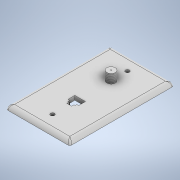
# Autodesk Inventor part: ethernet_coax_plug
Saved by Autodesk Inventor 2022 (Build 260153000, 153)
## iProperties
Created: 2022-01-23
Part Number: ethernet_coax_plug
Material: Generic
Document SubType Name: Modeling
Designer: kylem
Density: 1 g/cm^3
Appearance: Default
Author: kylem
Autodesk Inventor part; units mm, degrees
ref_plane "YZ Plane" through (0, 0, 0) normal (1, 0, 0) x (0, 1, 0)
ref_plane "XZ Plane" through (0, 0, 0) normal (0, 1, 0) x (-1, 0, 0)
ref_plane "XY Plane" through (0, 0, 0) normal (0, 0, 1) x (1, 0, 0)
sketch "Sketch1" plane through (0, 0, 0) normal (0, 1, 0) x (-1, 0, 0)
  line L0 (0, 0) -> (70, 0)
  line L1 (70, 0) -> (70, -114.4)
  line L2 (70, -114.4) -> (0, -114.4)
  line L3 (0, -114.4) -> (0, 0)
  dimension "d0" = 70
  dimension "d1" = 114.4
  constraints: 8 end point, 2 parallel, 1 horizontal, 1 perpendicular
  measures "d0" distance of L1.end L2.end
  measures "d1" distance of L0.end L1.end
extrude "Extrusion1" add sketch "Sketch1" along normal blind 4.65
sketch "Sketch2" plane through (0, 4.65, 0) normal (0, 1, 0) x (1, 0, 0)
  line L0 (-70, 0) -> (0, 0) projected
  line L1 (0, 0) -> (-35, 0)
  line L2 (-35, 0) -> (-35, 16)
  circle A0 centre (-35, 16) radius 2.125
  line L3 (0, 0) -> (0, 114.4) projected
  line L4 (0, 0) -> (0, 114.4)
  line L5 (0, 57.2) -> (13.6816, 57.2)
  circle A1 centre (-35, 98.4) radius 2.125
  dimension "d4" = 35
  dimension "d5" = 16
  dimension "d6" = 90
  dimension "d7" = 4.25
  constraints: 8 end point, 2 centre point, 2 midpoint, 1 coincident, 1 collinear, 1 horizontal, 1 perpendicular, 1 symmetric about line, 1 other
  measures "d4" distance of L0.end L1.end
  measures "d5" distance of L1.end L2.end
  measures "d6" angle of L1 L2
  measures "d7" diameter of A0
extrude "Extrusion2" cut sketch "Sketch2" against normal blind 10
fillet "Fillet1" radius 4.65 4 edges at (-35, 4.65, -114.4) (0, 4.65, -57.2) (-35, 4.65, 0) (-70, 4.65, -57.2)
fillet "Fillet2" radius 2 4 edges at (-1.3618, 3.2882, -1.3618) (-68.6382, 3.2882, -1.3618) (-68.6382, 3.2882, -113.0382) (-1.3618, 3.2882, -113.0382)
sketch "Sketch3" plane through (0, 4.65, 0) normal (0, 1, 0) x (1, 0, 0)
  line L0 (0, 0) -> (0, 34.4)
  line L1 (0, 2) -> (0, 112.4) projected
  line L2 (0, 34.4) -> (-70, 34.4)
  line L3 (-70, 112.4) -> (-70, 2) projected
  line L4 (-35, 34.4) -> (-29.125, 34.4)
  line L5 (-29.125, 34.4) -> (-40.875, 34.4)
  line L6 (-40.875, 34.4) -> (-40.875, 46.4)
  line L7 (-40.875, 46.4) -> (-29.125, 46.4)
  line L8 (-29.125, 46.4) -> (-29.125, 34.4)
  line L9 (-35, 34.4) -> (-32.34, 34.4)
  line L10 (-32.34, 34.4) -> (-32.34, 36.9)
  line L11 (-32.34, 36.9) -> (-31.09, 36.9)
  line L12 (-31.09, 36.9) -> (-31.09, 38.9)
  line L13 (-31.09, 38.9) -> (-28.2521, 38.9)
  line L14 (-35, 34.4) -> (-35, 32.315)
  line L15 (-37.66, 34.4) -> (-37.66, 36.9)
  line L16 (-37.66, 36.9) -> (-38.91, 36.9)
  line L17 (-38.91, 36.9) -> (-38.91, 38.9)
  line L18 (-38.91, 38.9) -> (-41.7479, 38.9)
  point P0 (-40.875, 38.9)
  point P1 (-29.125, 38.9)
  dimension "d12" = 34.4
  dimension "d13" = 70
  dimension "d14" = 5.875
  dimension "d15" = 11.75
  dimension "d16" = 12
  dimension "d17" = 2.66
  dimension "d18" = 2.5
  dimension "d19" = 1.25
  dimension "d20" = 2
  constraints: 34 end point, 5 symmetric about line, 4 perpendicular, 4 point on line, 2 horizontal, 2 parallel, 1 midpoint, 1 vertical
  measures "d12" distance of L0.start L0.end
  measures "d13" distance of L0.end L2.end
  measures "d14" distance of L4.start L4.end
  measures "d15" distance of L6.end L7.end
  measures "d16" distance of L5.end L6.end
  measures "d17" distance of L4.start L9.end
  measures "d18" distance of L9.end L10.end
  measures "d19" distance of L10.end L11.end
  measures "d20" distance of L11.end L12.end
extrude "Extrusion3" cut sketch "Sketch3" against normal blind 10 contours L2 L15 L16 L17 L18 L6 L7 L8 L13 L12 L11 L10
sketch "Sketch4" plane through (0, 4.65, 0) normal (0, 1, 0) x (1, 0, 0)
  line L0 (0, 0) -> (0, 114.4)
  line L1 (0, 2) -> (0, 112.4) projected
  line L2 (0, 114.4) -> (-35, 114.4)
  line L3 (-2, 114.4) -> (-68, 114.4) projected
  line L4 (-35, 114.4) -> (-35, 80.4)
  circle A0 centre (-35, 80.4) radius 4.625
  dimension "d23" = 114.4
  dimension "d24" = 34
  dimension "d25" = 9.25
  constraints: 6 end point, 1 centre point, 1 coincident, 1 collinear, 1 midpoint, 1 perpendicular
  measures "d23" distance of L0.start L0.end
  measures "d24" distance of L2.end L4.end
  measures "d25" diameter of A0
extrude "Extrusion4" add sketch "Sketch4" along normal blind 10
thread "Thread1" size "M10x1.5" class "6g" standard "ANSI Metric M Profile" full length
sketch "Sketch5" plane through (-35, 14.65, -80.4) normal (0, 1, 0) x (1, 0, 0)
  circle A0 centre (0, 0) radius 0.5
  point P0 (35, -80.4)
  dimension "d30" = 1
  constraints: 1 centre point
  measures "d30" diameter of A0
extrude "Extrusion5" cut sketch "Sketch5" against normal blind 3
body "Solid1"
